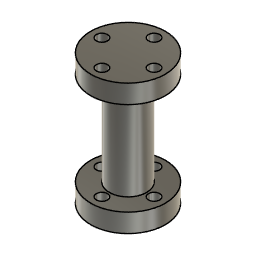
Offset Joint v4 (Autodesk Fusion 360 design; units mm, degrees)
Autodesk Fusion 360 part; units mm, degrees
sketch "Sketch1" plane through (0, 0, 0) normal (0, 0, 1) x (1, 0, 0)
  circle A0 centre (0, 0) radius 7 construction
  circle A1 centre (-7, 0) radius 1.5
  circle A2 centre (0, 7) radius 1.5
  circle A3 centre (7, 0) radius 1.5
  circle A4 centre (0, -7) radius 1.5
  circle A5 centre (0, 0) radius 10
  circle A6 centre (0, 0) radius 5
  dimension "d5" = 360
  dimension "d7" = 14
  dimension "d8" = 3
  dimension "d11" = 20
  dimension "d15" = 10
  constraint coincident A2.centre A0
  constraint vertical A2.centre A0.centre
  constraint coincident A0.centre A5.centre
  constraint concentric A0 A5
  constraint concentric A0 A6
  measures "d7" diameter of A0
  measures "d8" diameter of A2
  measures "d11" diameter of A5
  measures "d15" diameter of A6
extrude "Extrude1" add sketch "Sketch1" along normal blind 5 contours A5 | A6
extrude "Extrude2" add sketch "Sketch1" against normal blind 30 contours A6
sketch "Sketch3" plane through (0, 0, -30) normal (0, 0, -1) x (1, 0, 0)
  circle A0 centre (0, 0) radius 5
  circle A1 centre (0, 7) radius 1.5
  circle A2 centre (0, 0) radius 5
  circle A3 centre (0, 0) radius 7 construction
  circle A4 centre (-7, 0) radius 1.5
  circle A5 centre (0, -7) radius 1.5
  circle A6 centre (7, 0) radius 1.5
  circle A7 centre (0, 0) radius 10
  dimension "d20" = 360
  dimension "d21" = 14
  dimension "d22" = 3
  dimension "d23" = 20
  dimension "d24" = 10
  constraint coincident A1.centre A3
  constraint vertical A1.centre A0.centre
  constraint coincident A0.centre A2.centre
  constraint concentric A3 A7
  constraint concentric A2 A3
  measures "d21" diameter of A3
  measures "d22" diameter of A1
  measures "d23" diameter of A7
  measures "d24" diameter of A2
extrude "Extrude4" add sketch "Sketch3" against normal blind 5
equation "outer_radius = 20 mm"
equation "radius_thickness = 5 mm"
equation "d11 = outer_radius"
equation "d12 = radius_thickness"
equation "inner_radius = 10 mm"
equation "d15 = inner_radius"
equation "tot_height = 35 mm"
equation "d17 = -tot_height + radius_thickness"
equation "d23 = outer_radius"
equation "d24 = inner_radius"
equation "d27 = -radius_thickness"
